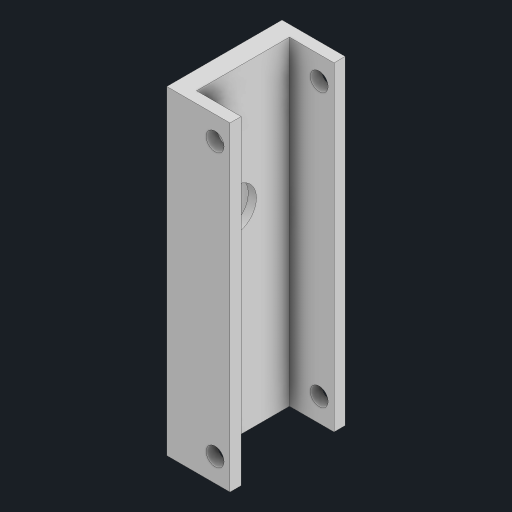
# Autodesk Inventor part: TH_fan_holder
Saved by Autodesk Inventor 2024.1 (Build 281209000, 209)
## iProperties
Created: 2024-08-15
Part Number: TH_fan_holder
Material: Generic
Document SubType Name: Modeling
Designer: luisg
Density: 1 g/cm^3
Appearance: Default
Author: luisg
Autodesk Inventor part; units mm, degrees
ref_plane "YZ Plane" through (0, 0, 0) normal (1, 0, 0) x (0, 1, 0)
ref_plane "XZ Plane" through (0, 0, 0) normal (0, 1, 0) x (-1, 0, 0)
ref_plane "XY Plane" through (0, 0, 0) normal (0, 0, 1) x (1, 0, 0)
sketch "Sketch1" plane through (0, 0, 0) normal (1, 0, 0) x (0, 1, 0)
  line L0 (43, 15.5) -> (-43, 15.5)
  line L1 (-43, 15.5) -> (-43, -15.5)
  line L2 (-43, -15.5) -> (43, -15.5)
  line L3 (43, -15.5) -> (43, 15.5)
  point P0 (0, 0)
  point P1 (0, -15.5)
  point P2 (43, 0)
  dimension "d0" = 86
  dimension "d1" = 31
  constraints: 8 end point, 3 perpendicular, 2 midpoint, 1 horizontal, 1 horizontal alignment, 1 vertical alignment
  measures "d0" distance of L1.end L2.end
  measures "d1" distance of L0.end L1.end
extrude "Extrusion1" add sketch "Sketch1" along normal blind 5
sketch "Sketch2" plane through (5, 0, 0) normal (1, 0, 0) x (0, 0, -1)
  line L0 (-15.5, 43) -> (-12.5, 43)
  line L1 (-12.5, 43) -> (-12.5, -43)
  line L2 (-12.5, -43) -> (-15.5, -43)
  line L3 (-15.5, -43) -> (-15.5, 43)
  line L4 (12.5, 43) -> (15.5, 43)
  line L5 (15.5, 43) -> (15.5, -43)
  line L6 (15.5, -43) -> (12.5, -43)
  line L7 (12.5, -43) -> (12.5, 43)
  point P0 (0, 0)
  dimension "d4" = 3
  dimension "d5" = 3
  constraints: 16 end point, 6 perpendicular, 4 coincident, 2 horizontal
  measures "d4" distance between parallel lines of L3 L1
  measures "d5" distance between parallel lines of L5 L7
extrude "Extrusion2" add sketch "Sketch2" along normal blind 12
sketch "Sketch3" plane through (0, -43, -15.5) normal (0, 0, -1) x (-1, 0, 0)
  line L0 (0, 86) -> (-17, 86) construction
  line L1 (-5, 0) -> (-5, 86) construction
  line L2 (-35.4485, 43) -> (35.4485, 43) construction
  line L3 (0, 0) -> (0, 86) construction
  point P0 (0, 43)
  point P1 (-13, 79.7)
  point P2 (0, 43)
  point P3 (-13, 6.3)
  dimension "d8" = 6.3
  dimension "d9" = 8
  constraints: 2 end point, 2 midpoint, 1 horizontal, 1 symmetric about line
  measures "d8" distance from line of L0 point (-13, 79.7)
  measures "d9" distance from line of L1 point (-13, 79.7)
hole "Hole1" at (13, 36.7, -15.5) at (13, -36.7, -15.5) direction (0, 0, 1) diameter 4.8 end through all
sketch "Sketch4" plane through (5, 0, 0) normal (1, 0, 0) x (0, 0, -1)
  line L0 (-15.5, 43) -> (-15.5, -43) projected
  point P0 (0, 0)
  point P1 (-2.1, 10)
  dimension "d25" = 13.4
  dimension "d26" = 10
  measures "d25" distance from line of L0 point (-2.1, 10)
  measures "d26" vertical distance of point (0, 0) point (-2.1, 10)
hole "Hole2" at (5, 10, 2.1) direction (-1, 0, 0) diameter 6.6 depth 5 counterbore diameter 11.4 counterbore depth 2.2 clearance for "Countersunk Flat Head Screw ISO 2009/7046" size "M6" standard "ISO"
body "Solid1"
